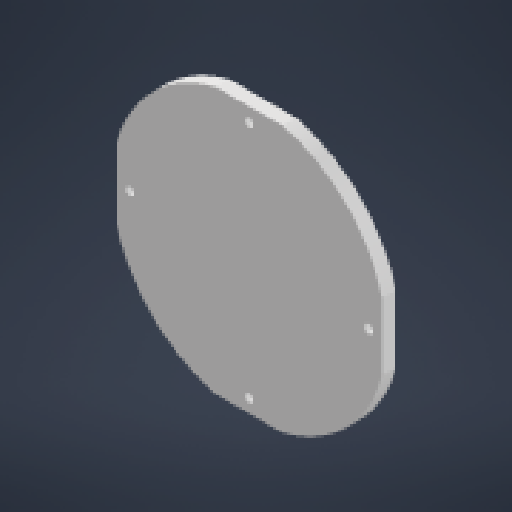
# Autodesk Inventor part: plate_lower
Saved by Autodesk Inventor 2027 (Build 310192000, 192)
## iProperties
Created: 2026-10-07
Part Number: plate_lower
Material: Generisch
Document SubType Name: Modeling
Designer: luca
Density: 1 g/cm^3
Appearance: Vorgabe
Author: luca
Autodesk Inventor part; units mm, degrees
ref_plane "YZ Plane" through (0, 0, 0) normal (1, 0, 0) x (0, 1, 0)
ref_plane "XZ Plane" through (0, 0, 0) normal (0, 1, 0) x (-1, 0, 0)
ref_plane "XY Plane" through (0, 0, 0) normal (0, 0, 1) x (1, 0, 0)
sketch "Skizze1" plane through (0, 0, 0) normal (0, 1, 0) x (-1, 0, 0)
  circle A0 centre (0, 0) radius 100
  dimension "d0" = 200
  constraints: 1 centre point, 1 coincident
  measures "d0" diameter of A0
extrude "Extrusion1" add sketch "Skizze1" along normal blind 10
sketch "Skizze2" plane through (0, 10, 0) normal (0, 1, 0) x (1, 0, 0)
  circle A0 centre (0, 0) radius 100 projected
  circle A1 centre (-87, 0) radius 3.1
  dimension "d3" = 6.2
  dimension "d4" = 87
  dimension "d5" = 200
  constraints: 1 centre point, 1 horizontal alignment
  measures "d3" diameter of A1
  measures "d4" distance of A1.centre A0.centre
  measures "d5" diameter of A0
extrude "Extrusion2" cut sketch "Skizze2" against normal through all contours A1
sketch "Skizze3" plane through (0, 10, 0) normal (0, 1, 0) x (1, 0, 0)
  circle A0 centre (-87, 0) radius 3.1 projected
  circle A1 centre (0, 0) radius 100 projected
  line L0 (-97, -24.3105) -> (-97, 24.3105)
  circle A2 centre (0, 0) radius 100 projected
  point P0 (-97, -24.3105)
  dimension "d11" = 10
  constraints: 2 end point, 1 point on circle, 1 vertical, 2 other
  measures "d11" distance from line of A0.centre L0
extrude "Extrusion3" cut sketch "Skizze3" against normal through all contours L0 A1 picked at (-97.7491, 4.0825)
pattern_circular "Runde Anordnung3" count 4 over 360 about axis through (0, -10, 0) along (0, 1, 0) of "Extrusion2"
pattern_circular "Runde Anordnung4" count 4 over 360 about axis through (0, -10, 0) along (0, 1, 0) of "Extrusion3"
chamfer "Fasen2" distance 4 angle 45 4 edges at (-90.1, 10, 0) (0, 10, -90.1) (90.1, 10, 0) (0, 10, 90.1)
